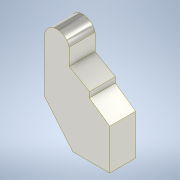
# Autodesk Inventor part: McCrea_velky_krk_walle
Saved by Autodesk Inventor 2022 (Build 260153000, 153)
## iProperties
Created: 2022-01-10
Part Number: McCrea_velky_krk_walle
Material: Generic
Document SubType Name: Modeling
Designer: student
Density: 1 g/cm^3
Appearance: Silver
Author: student
Autodesk Inventor part; units mm, degrees
ref_plane "YZ Plane" through (0, 0, 0) normal (1, 0, 0) x (0, 1, 0)
ref_plane "XZ Plane" through (0, 0, 0) normal (0, 1, 0) x (-1, 0, 0)
ref_plane "XY Plane" through (0, 0, 0) normal (0, 0, 1) x (1, 0, 0)
sketch "Sketch1" plane through (0, 0, 0) normal (0, 0, 1) x (1, 0, 0)
  line L0 (-21.9931, 0) -> (-11.9931, 0)
  line L1 (-11.9931, 0) -> (-11.9931, 11)
  line L2 (-21.9931, 0) -> (-29.7066, 9.1925)
  line L3 (-29.7066, 9.1925) -> (-29.7066, 23.1925)
  line L4 (-11.9931, 11) -> (-17.4931, 14.8511)
  line L5 (-17.4931, 14.8511) -> (-17.4931, 16.3511)
  line L6 (-17.4931, 16.3511) -> (-22.9931, 19.5266)
  line L7 (-22.9931, 19.5266) -> (-22.9931, 24.0266)
  arc A0 (-22.9931, 24.0266) -> (-29.7066, 23.1925) centre (-26.298, 23.1925) ccw
  line L8 (-36.09, 0) -> (6.015, 0) projected
  point P0 (0, 0)
  dimension "d0" = 10
  dimension "d1" = 11
  dimension "d2" = 5.5
  dimension "d4" = 5.5
  dimension "d5" = 12
  dimension "d6" = 14
  dimension "d7" = 1.5
  dimension "d9" = 130
  dimension "d10" = 125
  dimension "d12" = 4.5
  dimension "d13" = 120
  constraints: 16 end point, 2 point on circle, 2 vertical, 1 centre point, 1 collinear, 1 parallel, 1 perpendicular, 1 tangent
  measures "d0" distance of L0.start L0.end
  measures "d1" distance of L0.end L1.end
  measures "d2" horizontal distance of L1.end L4.end
  measures "d4" horizontal distance of L5.end L6.end
  measures "d5" distance of L0.start L2.end
  measures "d6" distance of L2.end L3.end
  measures "d7" distance of L4.end L5.end
  measures "d9" angle of L0 L2
  measures "d10" angle of L1 L4
  measures "d12" distance of L6.end L7.end
  measures "d13" angle of L5 L6
extrude "Extrusion1" add sketch "Sketch1" along normal blind 7
sketch "Sketch3" plane through (-21.9931, 0, 0) normal (0, -1, 0) x (1, 0, 0)
  circle A0 centre (5, 3.5) radius 1.5
  line L0 (0, 7) -> (10, 7) projected
  line L1 (10, 0) -> (10, 7) projected
  line L2 (0, 0) -> (0, 7) projected
  point P0 (21.9931, 0)
  dimension "d23" = 3.5
  dimension "d24" = 5
  dimension "d33" = 3
  constraints: 1 centre point
  measures "d23" distance from line of L0 A0.centre
  measures "d24" distance from line of L1 A0.centre
  measures "d33" diameter of A0
hole "Hole2" at (-16.9931, 0, 3.5) direction (0, 1, 0) diameter 3 depth 3 tip angle 118
body "Solid1"
